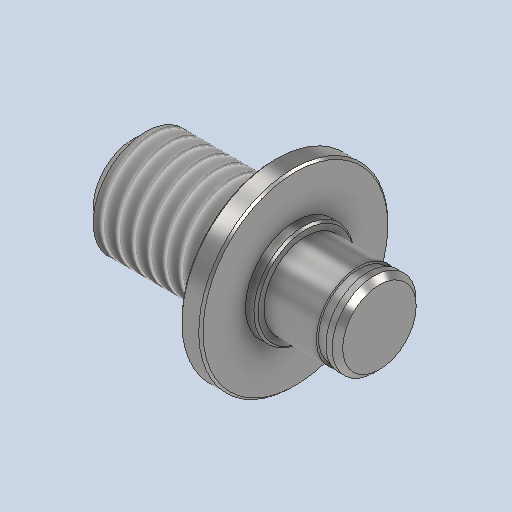
# Autodesk Inventor part: ParallelMech_SupportLink_Distall_JointShaft
Saved by Autodesk Inventor 2024 (Build 280153000, 153)
## iProperties
Created: 2022-07-30
Part Number: ParallelMech_SupportLink_Distall_JointShaft
Material: Edelstahl
Document SubType Name: Modeling
Designer: alexw
Density: 8 g/cm^3
Appearance: Halbpoliert
Mass: 15.6737 g
Surface Area: 12.1097 cm^2
Volume: 1.95921 cm^3
JTM_1018_Thickness: 1,000 mm
Bearing_Flansch_Thickness: 1,100 mm
Bearing_Thickness: 5,000 mm
Author: alexw
Autodesk Inventor part; units mm, degrees
ref_plane "YZ Plane" through (0, 0, 0) normal (1, 0, 0) x (0, 1, 0)
ref_plane "XZ Plane" through (0, 0, 0) normal (0, 1, 0) x (-1, 0, 0)
ref_plane "XY Plane" through (0, 0, 0) normal (0, 0, 1) x (1, 0, 0)
sketch "Skizze1" plane through (0, 0, 0) normal (0, 0, 1) x (1, 0, 0)
  line L0 (0, 0) -> (0, 4.75)
  line L1 (0, 4.75) -> (3, 4.75)
  line L2 (3, 4.75) -> (3, 4)
  line L3 (3, 4) -> (8, 4)
  line L4 (8, 4) -> (8, 3.8)
  line L5 (8, 3.8) -> (8.9, 3.8)
  line L6 (8.9, 3.8) -> (8.9, 4)
  line L7 (8.9, 4) -> (9.5, 4)
  line L8 (10, 3.5) -> (10, 0)
  line L9 (10, 0) -> (0, 0)
  line L10 (0, 5) -> (-12.25, 5)
  line L11 (-13.5, 3.75) -> (-13.5, 0)
  line L12 (-13.5, 0) -> (0, 0)
  line L13 (9.5, 4) -> (10, 3.5)
  line L14 (-13.5, 3.75) -> (-12.25, 5)
  line L15 (8, 4) -> (8, 0) construction
  line L16 (2, 4.75) -> (2, 9)
  line L17 (2, 9) -> (0, 9)
  line L18 (0, 9) -> (0, 4.75)
  line L19 (3, 4) -> (3, 0) construction
  point P0 (10, 4)
  point P1 (-13.5, 5)
  dimension "d0" = 7.6
  dimension "d1" = 0.5
  dimension "d2" = 0.5
  dimension "d3" = 0.9
  dimension "d4" = 8
  dimension "d5" = 0.6
  dimension "d6" = 9.5
  dimension "d8" = 10
  dimension "d9" = 1.25
  dimension "d10" = 1.25
  dimension "d11" = 13.5
  dimension "d15" = 0
  dimension "d22" = 1
  dimension "d23" = 18
  dimension "d24" = 5
  dimension "d25" = 0
  dimension "d27" = 3
  constraints: 40 end point, 14 perpendicular, 12 point on line, 2 vertical, 1 collinear
  measures "d0" diameter of L5 L9
  measures "d1" distance of L7.end point (10, 4)
  measures "d2" distance of L8.start point (10, 4)
  measures "d3" distance between parallel lines of L6 L4
  measures "d4" diameter of L3 L9
  measures "d5" distance from line of L7.end L6
  measures "d6" diameter of L1 L9
  measures "d8" diameter of L10 L12
  measures "d9" distance of L11.start point (-13.5, 5)
  measures "d10" distance of L10.end point (-13.5, 5)
  measures "d11" distance between parallel lines of L0 L11
  measures "d15" distance from line of L15 L3.end
  measures "d22" distance between parallel lines of L2 L16
  measures "d23" diameter of L17 L9
  measures "d24" distance between parallel lines of L15 L19
  measures "d25" distance between parallel lines of L19 L2
  measures "d27" distance between parallel lines of L19 L0
revolve "Umdrehung1" add sketch "Skizze1" angle 360 about axis through (10, 0, 0) along (-1, 0, 0)
thread "Gewinde1" size "M10x1.5" class "6g" standard "ANSI Metric M Profile" full length
chamfer "Fase1" distance 0.2 angle 45 3 edges at (3, -4.75, 0) (2, -9, 0) (0, -9, 0)
equation "\"d2\" = d1"
equation "\"d10\" = d9"
equation "\"d22\" = JTM_1018_Thickness"
equation "\"d24\" = Bearing_Thickness"
equation "\"Bearing_StepThickness\" = 2"
equation "\"SupportLink_Bearing_StepDia\" = 13"
equation "\"Bearing_Thickness\" = 5"
equation "\"Bearing_Flansch_Thickness\" = 1.1"
equation "\"JTM_1018_Thickness\" = 1"
